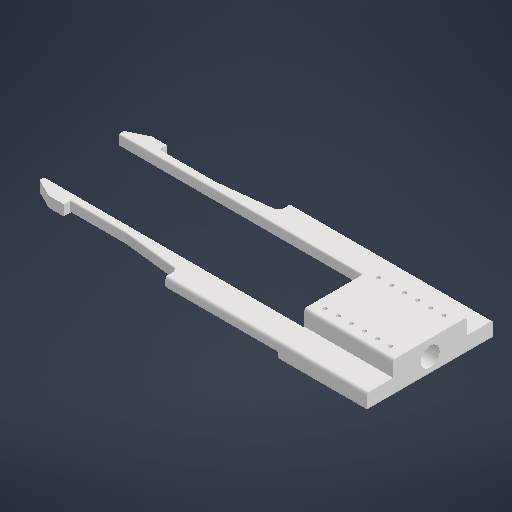
# Autodesk Inventor part: Tourniquet_Rail_01_V4
Saved by Autodesk Inventor 2026.2 (Build 302298000, 298)
## iProperties
Created: 2026-03-17
Part Number: Tourniquet_Rail_01_V4
Material: Generic
Document SubType Name: Modeling
Designer: vckot
Density: 1 g/cm^3
Appearance: Default
Author: vckot
Autodesk Inventor part; units mm, degrees
ref_plane "YZ Plane" through (0, 0, 0) normal (1, 0, 0) x (0, 1, 0)
ref_plane "XZ Plane" through (0, 0, 0) normal (0, 1, 0) x (-1, 0, 0)
ref_plane "XY Plane" through (0, 0, 0) normal (0, 0, 1) x (1, 0, 0)
sketch "Sketch1" plane through (0, 0, 0) normal (1, 0, 0) x (0, 1, 0)
  line L0 (-5, 0) -> (5, 0) construction
  line L1 (-5, -14.125) -> (-5, 14.125)
  line L2 (0, -14.125) -> (-5, -14.125)
  arc A0 (0, -14.125) -> (4.125, -10) centre (0, -10) ccw
  line L3 (4.125, 10) -> (4.125, -10)
  arc A1 (4.125, 10) -> (0, 14.125) centre (0, 10) ccw
  line L4 (-5, 14.125) -> (0, 14.125)
  point P0 (0, 0)
  point P1 (-2.5, 14.125)
  point P2 (2.5, 13.2811)
  point P3 (-2.5, -14.125)
  point P4 (2.5, -13.2811)
  point P5 (4.125, 0)
  point P6 (0, 0)
  point P7 (-2.5, 20.8125)
  point P8 (-2.5, 14.125)
  point P9 (-2.5, -20.8125)
  point P10 (-2.5, -14.125)
  dimension "d8" = 10
  dimension "d17" = 9.125
  dimension "d18" = 28.25
  dimension "d19" = 4.125
  dimension "d20" = 4.125
  dimension "d59" = 5
  dimension "d60" = 14.125
  constraints: 10 end point, 6 midpoint, 6 point on circle, 4 tangent, 2 centre point, 2 horizontal alignment, 2 vertical alignment, 1 horizontal, 1 perpendicular
  measures "d8" distance of L0.start L0.end
  measures "d17" distance between parallel lines of L1 L3
  measures "d18" distance between parallel lines of L2 L4
  measures "d19" radius of A1
  measures "d20" radius of A0
  measures "d59" distance from line of L1 point (0, 0)
  measures "d60" distance from line of L2 point (0, 0)
extrude "Extrusion1" add sketch "Sketch1" along normal blind 34
sketch "Sketch5" plane through (34, 0, 0) normal (1, 0, 0) x (0, 0, -1)
  circle A0 centre (0, 1) radius 5
  line L0 (-14.125, -5) -> (14.125, -5) projected
  line L1 (-14.125, -5) -> (14.125, -5)
  line L2 (14.125, -5) -> (14.125, 7)
  line L3 (14.125, 7) -> (-14.125, 7)
  line L4 (-14.125, 7) -> (-14.125, -5)
  line L5 (-14.125, 0) -> (-14.125, -5) projected
  line L6 (14.125, -5) -> (14.125, 0) projected
  circle A1 centre (0, 1) radius 3.65
  line L7 (-14.125, -3) -> (-24.125, -3)
  line L8 (-24.125, -3) -> (-24.125, 1)
  line L9 (-24.125, 1) -> (-14.125, 1)
  line L10 (-14.125, 1) -> (-14.125, -3)
  line L11 (14.125, 1) -> (24.125, 1)
  line L12 (24.125, -3) -> (14.125, -3)
  line L13 (14.125, -3) -> (14.125, 1)
  line L14 (24.125, 1) -> (24.125, -3)
  point P0 (0, -4)
  point P1 (0, 6)
  point P2 (0, -5)
  point P3 (-12.125, -5)
  point P4 (12.125, -5)
  point P5 (-14.125, -3)
  point P6 (-14.125, 1)
  point P7 (14.125, -3)
  dimension "d54" = 10
  dimension "d55" = 1
  dimension "d56" = 1
  dimension "d63" = 7.3
  dimension "d69" = 10
  dimension "d70" = 4
  dimension "d71" = 10
  dimension "d72" = 4
  dimension "d73" = 2
  dimension "d74" = 2
  dimension "d75" = 48.25
  constraints: 24 end point, 4 collinear, 4 parallel, 3 horizontal, 3 vertical alignment, 2 centre point, 2 midpoint, 2 perpendicular, 2 point on circle, 1 coincident, 1 point on line, 1 vertical
  measures "d54" diameter of A0
  measures "d55" distance from line of L0 A0.start
  measures "d56" distance from line of L3 A0.end
  measures "d63" diameter of A1
  measures "d69" distance of L8.end L9.end
  measures "d70" distance of L7.end L8.end
  measures "d71" distance of L12.start L12.end
  measures "d72" distance of L11.end L12.start
  measures "d73" distance between parallel lines of L0 L7
  measures "d74" distance between parallel lines of L0 L12
  measures "d75" distance between parallel lines of L14 L8
extrude "Extrusion3" add sketch "Sketch5" against normal up to surface (34 mm away) contours A0 | L4 L3 L2 L0 | L7 L8 L9 L4 | L2 L11 L14 L12 | A1
extrude "Extrusion4" cut sketch "Sketch5" against normal through all contours A1
sketch "Sketch6" plane through (0, 0, 0) normal (-1, 0, 0) x (0, 0, 1)
  circle A0 centre (0, 1) radius 5 projected
  point P0 (0, 0)
extrude "Extrusion5" cut sketch "Sketch6" against normal blind 10
sketch "Sketch3" plane through (34, 0, 0) normal (1, 0, 0) x (0, 0, -1)
  line L0 (-14.125, -5) -> (14.125, -5) projected
  line L1 (-14.125, -5) -> (-5.125, -5)
  line L2 (-5.125, -5) -> (-5.125, -2.5)
  line L3 (-5.125, -2.5) -> (-14.125, -2.5)
  line L4 (-14.125, -2.5) -> (-14.125, -5)
  line L5 (14.125, -5) -> (5.125, -5)
  line L6 (5.125, -5) -> (5.125, -2.5)
  line L7 (5.125, -2.5) -> (14.125, -2.5)
  line L8 (14.125, -2.5) -> (14.125, -5)
  point P0 (0, 0)
  dimension "d35" = 9
  dimension "d36" = 2.5
  dimension "d37" = 9
  dimension "d38" = 2.5
  constraints: 16 end point, 4 parallel, 2 horizontal, 2 perpendicular
  measures "d35" distance of L3.end L2.end
  measures "d36" distance of L2.end L1.end
  measures "d37" distance of L6.end L7.end
  measures "d38" distance of L5.end L6.end
extrude "Extrusion2" [suppressed]
sketch "Sketch4" plane through (34, -2.5, 14.125) normal (0, 1, 0) x (1, 0, 0)
  line L0 (21, 3.25) -> (4, 3.25) construction
  line L1 (21, 25) -> (4, 25) construction
  line L2 (0, 19.25) -> (25, 19.25) construction
  line L3 (0, 9) -> (25, 9) construction
  line L4 (25, 9) -> (25, 0) construction
  line L5 (25, 28.25) -> (25, 19.25) construction
  circle A0 centre (21, -4.25) radius 0.75 projected
  circle A1 centre (4, -4.25) radius 0.75 projected
  circle A2 centre (21, 32.5) radius 0.75 projected
  circle A3 centre (4, 32.5) radius 0.75 projected
  point P0 (-34, 14.125)
  point P1 (12.5, 25)
  point P2 (12.5, 19.25)
  point P3 (12.5, 3.25)
  point P4 (12.5, 9)
  dimension "d48" = 17
  dimension "d49" = 17
  dimension "d50" = 7.5
  dimension "d51" = 7.5
  constraints: 4 end point, 4 midpoint, 2 horizontal, 2 horizontal alignment, 2 vertical alignment
  measures "d48" distance of L0.start L0.end
  measures "d49" distance of L1.end L1.start
  measures "d50" distance of A2.centre L1.start
  measures "d51" distance of A0.centre L0.start
hole "Hole2" [suppressed]
fillet "Fillet1" [suppressed]
sketch "Sketch8" plane through (0, 1, 14.125) normal (0, 1, 0) x (1, 0, 0)
  line L0 (0, -10) -> (-65, -10)
  line L1 (-65, -10) -> (-65, 0)
  line L2 (-65, 0) -> (0, 0)
  line L3 (0, 0) -> (0, -10)
  line L4 (0, 38.25) -> (-65, 38.25)
  line L5 (-65, 38.25) -> (-65, 28.25)
  line L6 (-65, 28.25) -> (0, 28.25)
  line L7 (0, 28.25) -> (0, 38.25)
  line L8 (-65, 0) -> (-92, 0)
  line L9 (-92, 0) -> (-92, -2)
  line L10 (-90.3571, -3) -> (-65, -3)
  line L11 (-65, -3) -> (-65, 0)
  line L12 (0, 0) -> (0, 28.25) projected
  line L13 (-92, -2) -> (-86.25, -5.5)
  line L14 (-86.25, -5.5) -> (-86.25, -3)
  line L15 (0, 14.125) -> (-100.8608, 14.125) construction
  line L16 (-65, 28.25) -> (-92, 28.25)
  line L17 (-92, 28.25) -> (-92, 30.25)
  line L18 (-90.3571, 31.25) -> (-65, 31.25)
  line L19 (-92, 30.25) -> (-86.25, 33.75)
  line L20 (-86.25, 33.75) -> (-86.25, 31.25)
  point P0 (-75, -3)
  point P1 (-75, 31.25)
  dimension "d76" = 65
  dimension "d77" = 10
  dimension "d78" = 65
  dimension "d79" = 10
  dimension "d84" = 27
  dimension "d85" = 5.75
  dimension "d86" = 2
  dimension "d87" = 5.5
  dimension "d88" = 3
  dimension "d90" = 2.5
  constraints: 40 end point, 9 symmetric about line, 6 parallel, 5 point on line, 4 coincident, 4 horizontal, 4 perpendicular
  measures "d76" distance of L1.end L2.end
  measures "d77" distance of L0.end L1.end
  measures "d78" distance of L6.end L5.end
  measures "d79" distance of L5.end L4.end
  measures "d84" distance between parallel lines of L11 L9
  measures "d85" distance between parallel lines of L14 L9
  measures "d86" distance from line of L8 point (-92, -2)
  measures "d87" distance from line of L8 L13.end
  measures "d88" distance between parallel lines of L8 L10
  measures "d90" distance from line of L10 point (-86.25, -5.5)
extrude "Extrusion6" add sketch "Sketch8" against normal up to surface (4 mm away)
sketch "Sketch7" plane through (0, 1, 14.125) normal (0, 1, 0) x (1, 0, 0)
  line L0 (-65, -3) -> (-43, -5.5)
  line L1 (-43, -5.5) -> (-43, -10)
  line L2 (34, -10) -> (-65, -10) projected
  line L3 (-65, -3) -> (-65, -10) projected
  line L4 (34, 0) -> (34, 28.25) construction
  line L5 (34, 14.125) -> (-104.6483, 14.125) construction
  line L6 (-65, 31.25) -> (-43, 33.75)
  line L7 (-43, 33.75) -> (-43, 38.25)
  line L8 (-65, 31.25) -> (-65, 38.25)
  line L9 (34, -10) -> (-65, -10) projected
  line L10 (-65, 38.25) -> (-65, 31.25) projected
  line L11 (34, 38.25) -> (-65, 38.25) projected
  point P0 (0, 14.125)
  point P1 (-86.25, -5.5)
  point P2 (-65, -6.5)
  point P3 (-65, 34.75)
  dimension "d114" = 22
  constraints: 12 end point, 5 symmetric about line, 2 midpoint, 1 horizontal, 1 horizontal alignment, 1 point on line, 1 vertical
  measures "d114" distance from line of point (-65, -6.5) L1
extrude "Extrusion9" cut sketch "Sketch7" against normal blind 10
chamfer "Chamfer1" [suppressed]
chamfer "Chamfer2" [suppressed]
fillet "Fillet7" radius 10 2 edges at (-65, -1, -17.125) (-65, -1, 17.125)
sketch "Sketch9" plane through (0, -5, -14.125) normal (0, -1, 0) x (1, 0, 0)
  line L0 (-92, 0) -> (0, 0) projected
  line L1 (34, -10) -> (34, 0) projected
  line L2 (0, 0) -> (34, 0)
  line L3 (34, 0) -> (34, -10)
  line L4 (34, -10) -> (0, -10)
  line L5 (0, -10) -> (0, 0)
  line L6 (34, 28.25) -> (0, 28.25) projected
  line L7 (34, 38.25) -> (-43, 38.25) projected
  line L8 (0, 28.25) -> (34, 28.25)
  line L9 (34, 28.25) -> (34, 38.25)
  line L10 (34, 38.25) -> (0, 38.25)
  line L11 (0, 38.25) -> (0, 28.25)
  point P0 (0, 14.125)
  point P1 (-40, 38.25)
  point P2 (34, 0)
  point P3 (-65, 38.25)
  constraints: 16 end point, 4 parallel, 2 horizontal, 2 perpendicular
extrude "Extrusion7" add sketch "Sketch9" against normal up to surface (2 mm away)
sketch "Sketch10" plane through (-92, -3, 14.125) normal (0, -1, 0) x (1, 0, 0)
  line L0 (0, 2) -> (5.75, 5.5) projected
  line L1 (-7, 2) -> (-7, 0)
  line L2 (-7, 0) -> (0, 0)
  line L3 (0, 2) -> (5.75, 5.5) projected
  line L4 (0, 0) -> (0, 2) projected
  line L5 (0, -28.25) -> (-7, -28.25)
  line L6 (-7, -28.25) -> (-7, -30.25)
  line L7 (5.75, -31.25) -> (5.75, -33.75) projected
  line L8 (5.75, -33.75) -> (0, -30.25) projected
  line L9 (0, -30.25) -> (0, -28.25) projected
  line L10 (0, 0) -> (0, 2) projected
  line L11 (92, 0) -> (0, 0) projected
  line L12 (-7, -30.25) -> (0, -33.75)
  line L13 (0, -33.75) -> (5.75, -33.75)
  line L14 (-7, 2) -> (0, 5.5)
  line L15 (0, 5.5) -> (5.75, 5.5)
  point P0 (92, -14.125)
  point P1 (0, 1)
  dimension "d106" = 2
  dimension "d110" = 7
  dimension "d111" = 7
  dimension "d112" = 5.75
  dimension "d113" = 5.75
  constraints: 16 end point, 2 horizontal, 2 parallel, 2 perpendicular, 1 collinear, 1 midpoint
  measures "d106" distance of L5.end L6.end
  measures "d110" distance between parallel lines of L9 L6
  measures "d111" distance from line of point (0, 1) L1
  measures "d112" distance of L12.end L7.end
  measures "d113" distance of L14.end L0.end
extrude "Extrusion8" add sketch "Sketch10" against normal up to surface (4 mm away)
fillet "Fillet4" radius 1 10 edges at (-4.5, 1, 24.125) (-21.5, -3, 24.125) (-4.5, 1, -24.125) (-21.5, -3, -24.125) (17, 7, 14.125) (17, 7, -14.125) (34, -5, 0) (17, -5, 24.125) (0, -5, 0) (17, -5, -24.125)
fillet "Fillet5" radius 0.5 8 edges at (-49.5, 1, -14.125) (-49.5, -3, -14.125) (-49.5, 1, 14.125) (-49.5, -3, 14.125) (-75.9082, 1, 17.125) (-75.9082, -3, 17.125) (-75.9082, 1, -17.125) (-75.9082, -3, -17.125)
fillet "Fillet8" radius 2 6 edges at (-43, -2.8536, 19.4776) (-43, 0.8536, 19.4776) (-43, -1, 19.625) (-43, -2.8536, -19.4776) (-43, 0.8536, -19.4776) (-43, -1, -19.625)
sketch "Sketch11" plane through (34, 7, 13.125) normal (0, 1, 0) x (1, 0, 0)
  circle A0 centre (-5, 23.25) radius 0.75
  circle A1 centre (-5, 3) radius 0.75
  line L0 (0, 27.25) -> (-34, 27.25) projected
  line L1 (-34, -1) -> (0, -1) projected
  circle A2 centre (-10, 23.25) radius 0.75
  circle A3 centre (-10, 3) radius 0.75
  circle A4 centre (-15, 23.25) radius 0.75
  circle A5 centre (-15, 3) radius 0.75
  circle A6 centre (-20, 23.25) radius 0.75
  circle A7 centre (-20, 3) radius 0.75
  circle A8 centre (-25, 23.25) radius 0.75
  circle A9 centre (-25, 3) radius 0.75
  circle A10 centre (-30, 23.25) radius 0.75
  circle A11 centre (-30, 3) radius 0.75
  line L2 (0, 26.25) -> (0, 0) projected
  point P0 (-34, 13.125)
  dimension "d118" = 1.5
  dimension "d119" = 1.5
  dimension "d120" = 4
  dimension "d121" = 4
  dimension "d124" = 5
  dimension "d129" = 5
  constraints: 12 centre point, 1 horizontal, 1 vertical alignment, 20 other
  measures "d118" diameter of A0
  measures "d119" diameter of A1
  measures "d120" distance from line of L0 A0.centre
  measures "d121" distance from line of L1 A1.centre
  measures "d124" distance of A0.centre A2.centre
  measures "d129" distance from line of L2 A0.centre
extrude "Extrusion10" cut sketch "Sketch11" against normal through all
body "Solid1"
